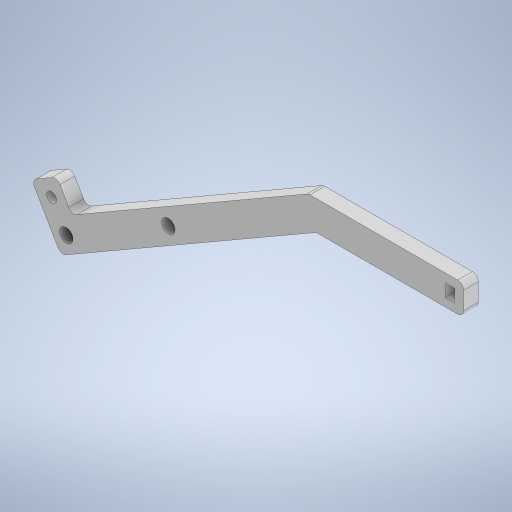
# Autodesk Inventor part: 刃固定パーツ
Saved by Autodesk Inventor 2024.3 (Build 283343000, 343)
## iProperties
Created: 2024-10-08
Part Number: 刃固定パーツ
Material: 一般
Document SubType Name: Modeling
Designer: hikou
Density: 1 g/cm^3
Appearance: 既定
Author: hikou
Autodesk Inventor part; units mm, degrees
ref_plane "YZ Plane" through (0, 0, 0) normal (1, 0, 0) x (0, 1, 0)
ref_plane "XZ Plane" through (0, 0, 0) normal (0, 1, 0) x (-1, 0, 0)
ref_plane "XY Plane" through (0, 0, 0) normal (0, 0, 1) x (1, 0, 0)
sketch "スケッチ1" plane through (0, 0, 0) normal (0, 0, 1) x (1, 0, 0)
  line L0 (0, 0) -> (52.6795, 0)
  line L1 (2.6795, -10) -> (52.6795, -10)
  line L2 (52.6795, 0) -> (52.6795, -10)
  line L3 (2.6795, -10) -> (-83.923, -60)
  line L4 (-80.2628, -46.3397) -> (0, 0)
  line L5 (-83.923, -60) -> (-93.923, -42.6795)
  line L6 (-93.923, -42.6795) -> (-85.2628, -37.6795)
  line L7 (-85.2628, -37.6795) -> (-80.2628, -46.3397)
  point P0 (-88.923, -51.3397)
  dimension "d1" = 50
  dimension "d2" = 10
  dimension "d3" = 100
  dimension "d4" = 150
  dimension "d5" = 10
  dimension "d6" = 20
  dimension "d7" = 10
  dimension "d8" = 10
  dimension "d9" = 10
  constraints: 16 end point, 2 horizontal, 2 perpendicular, 1 coincident, 1 midpoint, 1 parallel
  measures "d1" distance of L1.start L1.end
  measures "d2" distance of L0.end L1.end
  measures "d3" distance of L1.start L3.end
  measures "d4" angle of L1 L3
  measures "d5" distance between parallel lines of L4 L3
  measures "d6" distance of L3.end L5.end
  measures "d7" distance of L5.end L6.end
  measures "d8" distance of L4.start point (-88.923, -51.34)
  measures "d9" distance of L6.end L4.start
extrude "押し出し1" add sketch "スケッチ1" along normal mid plane 5
sketch "スケッチ2" plane through (0, 0, 2.5) normal (0, 0, 1) x (1, 0, 0)
  line L0 (46.4795, -7.1) -> (49.6795, -7.1)
  line L1 (49.6795, -7.1) -> (49.6795, -2.9)
  line L2 (49.6795, -2.9) -> (46.4795, -2.9)
  line L3 (46.4795, -2.9) -> (46.4795, -7.1)
  line L4 (46.4795, -7.1) -> (49.6795, -2.9) construction
  line L5 (49.6795, -7.1) -> (46.4795, -2.9) construction
  line L6 (52.6795, 0) -> (0, 0) projected
  line L7 (2.6795, -10) -> (52.6795, -10) projected
  line L8 (52.6795, -10) -> (52.6795, 0) projected
  point P0 (48.0795, -5)
  dimension "d14" = 3
  dimension "d15" = 3.2
  dimension "d41" = 4.2
  dimension "d42" = 2.9
  constraints: 12 end point, 2 midpoint, 2 parallel, 1 horizontal, 1 perpendicular
  measures "d14" distance between parallel lines of L8 L1
  measures "d15" distance between parallel lines of L1 L3
  measures "d41" distance of L0.end L1.end
  measures "d42" distance between parallel lines of L7 L0
extrude "押し出し2" cut sketch "スケッチ2" against normal blind 5
sketch "スケッチ3" plane through (0, 0, 2.5) normal (0, 0, 1) x (1, 0, 0)
  line L0 (-83.923, -60) -> (2.6795, -10) projected
  line L1 (-85.2628, -37.6795) -> (-93.923, -42.6795) projected
  line L2 (-80.2628, -46.3397) -> (-85.2628, -37.6795) projected
  line L3 (-93.923, -42.6795) -> (-83.923, -60) projected
  point P0 (0, 0)
  point P1 (-87.0929, -44.5096)
  point P2 (-82.0929, -53.1699)
  point P3 (-47.4519, -33.1699)
  dimension "d18" = 5
  dimension "d19" = 5
  dimension "d20" = 5
  dimension "d21" = 5
  dimension "d22" = 5
  dimension "d23" = 40
  measures "d18" distance from line of L0 point (-47.452, -33.17)
  measures "d19" distance from line of L0 point (-82.093, -53.17)
  measures "d20" distance from line of L1 point (-87.093, -44.51)
  measures "d21" distance from line of L2 point (-87.093, -44.51)
  measures "d22" distance from line of L3 point (-82.093, -53.17)
  measures "d23" distance of point (-47.452, -33.17) point (-82.093, -53.17)
hole "穴1" at (-82.0929, -53.1699, 2.5) at (-47.4519, -33.1699, 2.5) direction (0, 0, -1) diameter 4.5 end through all
fillet "フィレット1" radius 2 8 edges at (0, 0, 0) (2.6795, -10, 0) (52.6795, 0, 0) (52.6795, -10, 0) (-80.2628, -46.3397, 0) (-85.2628, -37.6795, 0) (-93.923, -42.6795, 0) (-83.923, -60, 0)
sketch "スケッチ4" plane through (0, 0, 2.5) normal (0, 0, 1) x (1, 0, 0)
  arc A0 (-84.923, -58.2679) -> (-82.191, -59) centre (-83.191, -57.2679) ccw projected
  line L0 (-82.191, -59) -> (2.2154, -10.2679) projected
  arc A1 (3.2154, -10) -> (2.2154, -10.2679) centre (3.2154, -12) ccw projected
  line L1 (3.2154, -10) -> (50.6795, -10) projected
  arc A2 (50.6795, -10) -> (52.6795, -8) centre (50.6795, -8) ccw projected
  line L2 (52.6795, -8) -> (52.6795, -2) projected
  arc A3 (52.6795, -2) -> (50.6795, 0) centre (50.6795, -2) ccw projected
  line L3 (50.6795, 0) -> (0.5359, 0) projected
  arc A4 (0.5359, 0) -> (-0.4641, -0.2679) centre (0.5359, -2) ccw projected
  line L4 (-0.4641, -0.2679) -> (-78.5307, -45.3397) projected
  arc A5 (-81.2628, -44.6077) -> (-78.5307, -45.3397) centre (-79.5307, -43.6077) ccw projected
  line L5 (-81.2628, -44.6077) -> (-84.2628, -39.4115) projected
  arc A6 (-84.2628, -39.4115) -> (-86.9948, -38.6795) centre (-85.9948, -40.4115) ccw projected
  line L6 (-86.9948, -38.6795) -> (-92.191, -41.6795) projected
  arc A7 (-92.191, -41.6795) -> (-92.923, -44.4115) centre (-91.191, -43.4115) ccw projected
  line L7 (-92.923, -44.4115) -> (-84.923, -58.2679) projected
  circle A8 centre (-47.4519, -33.1699) radius 2.25 projected
  circle A9 centre (-82.0929, -53.1699) radius 2.25 projected
  line L8 (46.4795, -2.9) -> (49.6795, -2.9) projected
  line L9 (49.6795, -2.9) -> (49.6795, -7.1) projected
  line L10 (49.6795, -7.1) -> (46.4795, -7.1) projected
  line L11 (46.4795, -7.1) -> (46.4795, -2.9) projected
  point P0 (0, 0)
  point P1 (-87.0929, -44.5096)
  dimension "d32" = 5
  dimension "d33" = 5
  measures "d32" distance from line of L5 point (-87.093, -44.51)
  measures "d33" distance from line of L6 point (-87.093, -44.51)
hole "穴2" at (-87.0929, -44.5096, 2.5) direction (0, 0, -1) diameter 3.3 end through all
equation "\"d19\" = d18"
equation "\"d20\" = d18"
equation "\"d21\" = d18"
equation "\"d22\" = d18"
